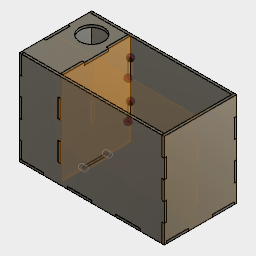
plant (Autodesk Fusion 360 design; units mm, degrees)
Autodesk Fusion 360 part; units mm, degrees
(part 1 of 2)
sketch "Sketch1" plane through (300, 0, 0) normal (1, 0, 0) x (0, 0, -1) in component "Right"
  line L0 (-145, 0) -> (-100, 0)
  line L1 (-100, 0) -> (-100, 5)
  line L2 (-100, 5) -> (-145, 5)
  line L3 (-145, 5) -> (-145, 0)
  line L4 (-50, 0) -> (-5, 0)
  line L5 (-5, 0) -> (-5, 5)
  line L6 (-5, 5) -> (-50, 5)
  line L7 (-50, 5) -> (-50, 0)
  line L8 (0, 0) -> (-150, 0)
  line L9 (-150, 0) -> (-150, 195)
  line L10 (-150, 195) -> (0, 195)
  line L11 (0, 195) -> (0, 0)
  dimension "d26" = 195
  measures "d26" distance of L8.end L9.end
extrude "Extrude1" add sketch "Sketch1" against normal blind 5 contours L1 L2 L3 L5 L6 L7 L8 L9 L10 L11 makes body 1 in component "Right"
sketch "Sketch2" plane through (300, 0, 0) normal (1, 0, 0) x (0, 0, -1) in component "Right"
  line L0 (0, 195) -> (-150, 195)
  line L1 (-150, 195) -> (-150, 0)
  line L2 (-150, 0) -> (-145, 0)
  line L3 (-145, 0) -> (-145, 5)
  line L4 (-145, 5) -> (-100, 5)
  line L5 (-100, 5) -> (-100, 0)
  line L6 (-100, 0) -> (-50, 0)
  line L7 (-50, 0) -> (-50, 5)
  line L8 (-50, 5) -> (-5, 5)
  line L9 (-5, 5) -> (-5, 0)
  line L10 (-5, 0) -> (0, 0)
  line L11 (0, 0) -> (0, 195)
  line L12 (-100, 195) -> (-100, 190)
  line L13 (-100, 190) -> (-145, 190)
  line L14 (-145, 190) -> (-145, 195)
  dimension "d29" = 5
  dimension "d30" = 45
  measures "d29" distance of L12.start L12.end
  measures "d30" distance of L12.end L13.end
extrude "Extrude2" cut sketch "Sketch2" against normal blind 5 contours L0 L12 L13 L14 bodies 1 in component "Right"
sketch "Sketch3" plane through (300, 0, 0) normal (1, 0, 0) x (0, 0, -1) in component "Right"
  line L0 (-145, 190) -> (-145, 195)
  line L1 (-145, 195) -> (-150, 195)
  line L2 (-150, 195) -> (-150, 0)
  line L3 (-150, 0) -> (-145, 0)
  line L4 (-145, 0) -> (-145, 5)
  line L5 (-145, 5) -> (-100, 5)
  line L6 (-100, 5) -> (-100, 0)
  line L7 (-100, 0) -> (-50, 0)
  line L8 (-50, 0) -> (-50, 5)
  line L9 (-50, 5) -> (-5, 5)
  line L10 (-5, 5) -> (-5, 0)
  line L11 (-5, 0) -> (0, 0)
  line L12 (0, 0) -> (0, 195)
  line L13 (0, 195) -> (-100, 195)
  line L14 (-100, 195) -> (-100, 190)
  line L15 (-100, 190) -> (-145, 190)
  line L16 (-50, 195) -> (-50, 190)
  line L17 (-50, 190) -> (-5, 190)
  line L18 (-5, 190) -> (-5, 195)
  line L19 (-50, 195) -> (-5, 195)
  dimension "d33" = 5
  dimension "d34" = 45
  measures "d33" distance of L16.start L16.end
  measures "d34" distance of L16.end L17.end
extrude "Extrude3" cut sketch "Sketch3" against normal blind 5 contours L13 L16 L17 L18 L19 bodies 1 in component "Right"
sketch "Sketch4" plane through (300, 0, 0) normal (1, 0, 0) x (0, 0, -1) in component "Right"
  line L0 (-50, 190) -> (-50, 195)
  line L1 (-50, 195) -> (-100, 195)
  line L2 (-100, 195) -> (-100, 190)
  line L3 (-100, 190) -> (-145, 190)
  line L4 (-145, 190) -> (-145, 195)
  line L5 (-145, 195) -> (-150, 195)
  line L6 (-150, 195) -> (-150, 0)
  line L7 (-150, 0) -> (-145, 0)
  line L8 (-145, 0) -> (-145, 5)
  line L9 (-145, 5) -> (-100, 5)
  line L10 (-100, 5) -> (-100, 0)
  line L11 (-100, 0) -> (-50, 0)
  line L12 (-50, 0) -> (-50, 5)
  line L13 (-50, 5) -> (-5, 5)
  line L14 (-5, 5) -> (-5, 0)
  line L15 (-5, 0) -> (0, 0)
  line L16 (0, 0) -> (0, 195)
  line L17 (0, 195) -> (-5, 195)
  line L18 (-5, 195) -> (-5, 190)
  line L19 (-5, 190) -> (-50, 190)
  line L20 (0, 0) -> (0, 39)
  line L21 (0, 39) -> (-5, 39)
  line L22 (-5, 39) -> (-5, 78)
  line L23 (-5, 78) -> (0, 78)
  dimension "d37" = 39
  dimension "d38" = 5
  dimension "d39" = 90
  dimension "d40" = 39
  dimension "d41" = 90
  dimension "d42" = 5
  measures "d37" distance of L15.end L20.end
  measures "d38" distance of L20.end L21.end
  measures "d39" angle of L21 L22
  measures "d40" distance of L21.end L22.end
  measures "d41" angle of L22 L23
  measures "d42" distance of L22.end L23.end
extrude "Extrude4" cut sketch "Sketch4" against normal blind 5 contours L16 L21 L22 L23 bodies 1 in component "Right"
sketch "Sketch5" plane through (300, 0, 0) normal (1, 0, 0) x (0, 0, -1) in component "Right"
  line L0 (0, 39) -> (-5, 39)
  line L1 (-5, 39) -> (-5, 78)
  line L2 (-5, 78) -> (0, 78)
  line L3 (0, 78) -> (0, 195)
  line L4 (0, 195) -> (-5, 195)
  line L5 (-5, 195) -> (-5, 190)
  line L6 (-5, 190) -> (-50, 190)
  line L7 (-50, 190) -> (-50, 195)
  line L8 (-50, 195) -> (-100, 195)
  line L9 (-100, 195) -> (-100, 190)
  line L10 (-100, 190) -> (-145, 190)
  line L11 (-145, 190) -> (-145, 195)
  line L12 (-145, 195) -> (-150, 195)
  line L13 (-150, 195) -> (-150, 0)
  line L14 (-150, 0) -> (-145, 0)
  line L15 (-145, 0) -> (-145, 5)
  line L16 (-145, 5) -> (-100, 5)
  line L17 (-100, 5) -> (-100, 0)
  line L18 (-100, 0) -> (-50, 0)
  line L19 (-50, 0) -> (-50, 5)
  line L20 (-50, 5) -> (-5, 5)
  line L21 (-5, 5) -> (-5, 0)
  line L22 (-5, 0) -> (0, 0)
  line L23 (0, 0) -> (0, 39)
  line L24 (0, 78) -> (0, 117)
  line L25 (0, 117) -> (-5, 117)
  line L26 (-5, 117) -> (-5, 156)
  line L27 (-5, 156) -> (0, 156)
  dimension "d45" = 39
  dimension "d46" = 5
  dimension "d47" = 90
  dimension "d48" = 39
  dimension "d49" = 90
  dimension "d50" = 5
  measures "d45" distance of L2.end L24.end
  measures "d46" distance of L24.end L25.end
  measures "d47" angle of L25 L26
  measures "d48" distance of L25.end L26.end
  measures "d49" angle of L26 L27
  measures "d50" distance of L26.end L27.end
extrude "Extrude5" cut sketch "Sketch5" against normal blind 5 contours L3 L25 L26 L27 bodies 1 in component "Right"
sketch "Sketch6" plane through (300, 0, 0) normal (1, 0, 0) x (0, 0, -1) in component "Right"
  line L0 (0, 117) -> (-5, 117)
  line L1 (-5, 117) -> (-5, 156)
  line L2 (-5, 156) -> (0, 156)
  line L3 (0, 156) -> (0, 195)
  line L4 (0, 195) -> (-5, 195)
  line L5 (-5, 195) -> (-5, 190)
  line L6 (-5, 190) -> (-50, 190)
  line L7 (-50, 190) -> (-50, 195)
  line L8 (-50, 195) -> (-100, 195)
  line L9 (-100, 195) -> (-100, 190)
  line L10 (-100, 190) -> (-145, 190)
  line L11 (-145, 190) -> (-145, 195)
  line L12 (-145, 195) -> (-150, 195)
  line L13 (-150, 195) -> (-150, 0)
  line L14 (-150, 0) -> (-145, 0)
  line L15 (-145, 0) -> (-145, 5)
  line L16 (-145, 5) -> (-100, 5)
  line L17 (-100, 5) -> (-100, 0)
  line L18 (-100, 0) -> (-50, 0)
  line L19 (-50, 0) -> (-50, 5)
  line L20 (-50, 5) -> (-5, 5)
  line L21 (-5, 5) -> (-5, 0)
  line L22 (-5, 0) -> (0, 0)
  line L23 (0, 0) -> (0, 39)
  line L24 (0, 39) -> (-5, 39)
  line L25 (-5, 39) -> (-5, 78)
  line L26 (-5, 78) -> (0, 78)
  line L27 (0, 78) -> (0, 117)
  line L28 (-150, 0) -> (-150, 39)
  line L29 (-150, 39) -> (-145, 39)
  line L30 (-145, 39) -> (-145, 78)
  line L31 (-145, 78) -> (-150, 78)
  line L32 (-150, 78) -> (-150, 117)
  line L33 (-150, 117) -> (-145, 117)
  line L34 (-145, 117) -> (-145, 156)
  line L35 (-145, 156) -> (-150, 156)
  dimension "d53" = 39
  dimension "d54" = 5
  dimension "d55" = 90
  dimension "d56" = 39
  dimension "d57" = 90
  dimension "d58" = 5
  dimension "d59" = 39
  dimension "d60" = 5
  dimension "d61" = 90
  dimension "d62" = 39
  measures "d53" distance of L13.end L28.end
  measures "d54" distance of L28.end L29.end
  measures "d55" angle of L29 L30
  measures "d56" distance of L29.end L30.end
  measures "d57" angle of L30 L31
  measures "d58" distance of L30.end L31.end
  measures "d59" distance of L31.end L32.end
  measures "d60" distance of L32.end L33.end
  measures "d61" angle of L33 L34
  measures "d62" distance of L33.end L34.end
extrude "Extrude6" cut sketch "Sketch6" against normal blind 5 contours L13 L33 L34 L35 | L13 L29 L30 L31 bodies 1 in component "Right"
sketch "Sketch7" plane through (295, 0, 0) normal (-1, 0, 0) x (0, 0, 1) in component "Right"
  line L0 (150, 117) -> (145, 117)
  line L1 (145, 117) -> (145, 156)
  line L2 (145, 156) -> (150, 156)
  line L3 (150, 156) -> (150, 195)
  line L4 (150, 195) -> (145, 195)
  line L5 (145, 195) -> (145, 190)
  line L6 (145, 190) -> (100, 190)
  line L7 (100, 190) -> (100, 195)
  line L8 (100, 195) -> (50, 195)
  line L9 (50, 195) -> (50, 190)
  line L10 (50, 190) -> (5, 190)
  line L11 (5, 190) -> (5, 195)
  line L12 (5, 195) -> (0, 195)
  line L13 (0, 195) -> (0, 156)
  line L14 (0, 156) -> (5, 156)
  line L15 (5, 156) -> (5, 117)
  line L16 (5, 117) -> (0, 117)
  line L17 (0, 117) -> (0, 78)
  line L18 (0, 78) -> (5, 78)
  line L19 (5, 78) -> (5, 39)
  line L20 (5, 39) -> (0, 39)
  line L21 (0, 39) -> (0, 0)
  line L22 (0, 0) -> (5, 0)
  line L23 (5, 0) -> (5, 5)
  line L24 (5, 5) -> (50, 5)
  line L25 (50, 5) -> (50, 0)
  line L26 (50, 0) -> (100, 0)
  line L27 (100, 0) -> (100, 5)
  line L28 (100, 5) -> (145, 5)
  line L29 (145, 5) -> (145, 0)
  line L30 (145, 0) -> (150, 0)
  line L31 (150, 0) -> (150, 39)
  line L32 (150, 39) -> (145, 39)
  line L33 (145, 39) -> (145, 78)
  line L34 (145, 78) -> (150, 78)
  line L35 (150, 78) -> (150, 117)
sketch "Sketch1 (2)" plane through (0, 0, 0) normal (-1, 0, 0) x (0, 0, 1) in component "Left"
  line L0 (100, 0) -> (150, 0)
  line L1 (150, 0) -> (150, 5)
  line L2 (150, 5) -> (100, 5)
  line L3 (100, 5) -> (100, 0)
  line L4 (0, 0) -> (50, 0)
  line L5 (50, 0) -> (50, 5)
  line L6 (50, 5) -> (0, 5)
  line L7 (0, 5) -> (0, 0)
  line L8 (150, 0) -> (0, 0)
  line L9 (0, 0) -> (0, 195)
  line L10 (0, 195) -> (150, 195)
  line L11 (150, 195) -> (150, 0)
  line L12 (100, 0) -> (100, 5)
  line L13 (100, 5) -> (145, 5)
  line L14 (145, 5) -> (145, 0)
  line L15 (5, 5) -> (5, 0)
  line L16 (150, 78) -> (145, 78)
  line L17 (145, 78) -> (145, 39)
  line L18 (145, 39) -> (150, 39)
  line L19 (150, 156) -> (145, 156)
  line L20 (145, 156) -> (145, 117)
  line L21 (145, 117) -> (150, 117)
  line L22 (100, 195) -> (100, 190)
  line L23 (100, 190) -> (145, 190)
  line L24 (145, 190) -> (145, 195)
  line L25 (50, 195) -> (50, 190)
  line L26 (50, 190) -> (5, 190)
  line L27 (5, 190) -> (5, 195)
  line L28 (0, 156) -> (5, 156)
  line L29 (5, 117) -> (0, 117)
  line L30 (5, 156) -> (5, 117)
  line L31 (0, 78) -> (5, 78)
  line L32 (5, 39) -> (0, 39)
  line L33 (5, 78) -> (5, 39)
  point P0 (0, 195)
  point P1 (145, 5)
  point P2 (145, 0)
  point P3 (5, 5)
  point P4 (5, 0)
  point P5 (150, 78)
  point P6 (145, 78)
  point P7 (145, 39)
  point P8 (150, 39)
  point P9 (150, 156)
  point P10 (145, 156)
  point P11 (145, 117)
  point P12 (150, 117)
  point P13 (100, 195)
  point P14 (100, 190)
  point P15 (145, 190)
  point P16 (145, 195)
  point P17 (50, 195)
  point P18 (50, 190)
  point P19 (5, 190)
  point P20 (5, 195)
  point P21 (0, 156)
  point P22 (5, 156)
  point P23 (5, 117)
  point P24 (0, 78)
  point P25 (5, 78)
  point P26 (5, 39)
extrude "Extrude1'" add sketch "Sketch1 (2)" against normal blind 5 separate body contours L2 L3 L5 L6 L8 L9 L10 L11 L12 L13 L16 L17 L18 L19 L20 L21 L22 L23 L24 L25 L26 L27 L28 L29 L30 L31 L32 L33 makes body 2 in component "Left"
sketch "Sketch1 (3)" plane through (0, 0, 0) normal (0, 0, -1) x (-1, 0, 0) in component "Back"
  line L0 (-250, 0) -> (-200, 0)
  line L1 (-200, 0) -> (-200, 5)
  line L2 (-200, 5) -> (-250, 5)
  line L3 (-250, 5) -> (-250, 0)
  line L4 (-150, 0) -> (-100, 0)
  line L5 (-100, 0) -> (-100, 5)
  line L6 (-100, 5) -> (-150, 5)
  line L7 (-150, 5) -> (-150, 0)
  line L8 (-50, 0) -> (0, 0)
  line L9 (0, 0) -> (0, 5)
  line L10 (0, 5) -> (-50, 5)
  line L11 (-50, 5) -> (-50, 0)
  line L12 (0, 5) -> (0, 39)
  line L13 (0, 39) -> (-5, 39)
  line L14 (-5, 39) -> (-5, 5)
  line L15 (-5, 5) -> (0, 5)
  line L16 (0, 78) -> (0, 117)
  line L17 (0, 117) -> (-5, 117)
  line L18 (-5, 117) -> (-5, 78)
  line L19 (-5, 78) -> (0, 78)
  line L20 (0, 156) -> (0, 195)
  line L21 (0, 195) -> (-5, 195)
  line L22 (-5, 195) -> (-5, 156)
  line L23 (-5, 156) -> (0, 156)
  line L24 (-300, 156) -> (-295, 156)
  line L25 (-295, 156) -> (-295, 195)
  line L26 (-295, 195) -> (-300, 195)
  line L27 (-300, 195) -> (-300, 156)
  line L28 (-295, 117) -> (-300, 117)
  line L29 (-300, 117) -> (-300, 78)
  line L30 (-300, 78) -> (-295, 78)
  line L31 (-295, 78) -> (-295, 117)
  line L32 (-295, 39) -> (-300, 39)
  line L33 (-300, 39) -> (-300, 0)
  line L34 (-300, 0) -> (-295, 0)
  line L35 (-295, 0) -> (-295, 39)
  line L36 (-300, 195) -> (0, 195)
  line L37 (0, 195) -> (0, 0)
  line L38 (0, 0) -> (-300, 0)
  line L39 (-300, 0) -> (-300, 195)
extrude "Extrude1''" add sketch "Sketch1 (3)" against normal blind 5 separate body contours L1 L2 L3 L5 L6 L7 L10 L11 L13 L14 L17 L18 L19 L22 L23 L24 L25 L28 L30 L31 L32 L35 L36 L37 L38 L39 makes body 3 in component "Back"
sketch "Sketch1 (4)" plane through (0, 0, 150) normal (0, 0, 1) x (1, 0, 0) in component "Front"
  line L0 (0, 0) -> (50, 0)
  line L1 (50, 0) -> (50, 5)
  line L2 (50, 5) -> (0, 5)
  line L3 (0, 5) -> (0, 0)
  line L4 (100, 0) -> (150, 0)
  line L5 (150, 0) -> (150, 5)
  line L6 (150, 5) -> (100, 5)
  line L7 (100, 5) -> (100, 0)
  line L8 (200, 0) -> (250, 0)
  line L9 (250, 0) -> (250, 5)
  line L10 (250, 5) -> (200, 5)
  line L11 (200, 5) -> (200, 0)
  line L12 (295, 156) -> (300, 156)
  line L13 (300, 156) -> (300, 195)
  line L14 (300, 195) -> (295, 195)
  line L15 (295, 195) -> (295, 156)
  line L16 (300, 117) -> (295, 117)
  line L17 (295, 117) -> (295, 78)
  line L18 (295, 78) -> (300, 78)
  line L19 (300, 78) -> (300, 117)
  line L20 (300, 39) -> (295, 39)
  line L21 (295, 39) -> (295, 0)
  line L22 (295, 0) -> (300, 0)
  line L23 (300, 0) -> (300, 39)
  line L24 (0, 39) -> (0, 5)
  line L25 (0, 5) -> (5, 5)
  line L26 (5, 5) -> (5, 39)
  line L27 (5, 39) -> (0, 39)
  line L28 (0, 117) -> (0, 78)
  line L29 (0, 78) -> (5, 78)
  line L30 (5, 78) -> (5, 117)
  line L31 (5, 117) -> (0, 117)
  line L32 (0, 195) -> (0, 156)
  line L33 (0, 156) -> (5, 156)
  line L34 (5, 156) -> (5, 195)
  line L35 (5, 195) -> (0, 195)
  line L36 (0, 195) -> (300, 195)
  line L37 (300, 195) -> (300, 0)
  line L38 (300, 0) -> (0, 0)
  line L39 (0, 0) -> (0, 195)
extrude "Extrude1'''" add sketch "Sketch1 (4)" against normal blind 5 separate body contours L1 L2 L5 L6 L7 L9 L10 L11 L12 L15 L16 L17 L18 L20 L21 L26 L27 L29 L30 L31 L33 L34 L36 L37 L38 L39 makes body 4 in component "Front"
sketch "Sketch2 (2)" plane through (300, 0, 0) normal (1, 0, 0) x (0, 0, -1) in component "Back"
  line L0 (-150, 156) -> (-145, 156)
  line L1 (-145, 156) -> (-145, 117)
  line L2 (-145, 117) -> (-150, 117)
  line L3 (-150, 117) -> (-150, 78)
  line L4 (-150, 78) -> (-145, 78)
  line L5 (-145, 78) -> (-145, 39)
  line L6 (-145, 39) -> (-150, 39)
  line L7 (-150, 39) -> (-150, 0)
  line L8 (-150, 0) -> (-145, 0)
  line L9 (-145, 0) -> (-145, 5)
  line L10 (-145, 5) -> (-100, 5)
  line L11 (-100, 5) -> (-100, 0)
  line L12 (-100, 0) -> (-50, 0)
  line L13 (-50, 0) -> (-50, 5)
  line L14 (-50, 5) -> (-5, 5)
  line L15 (-5, 5) -> (-5, 0)
  line L16 (-5, 0) -> (0, 0)
  line L17 (0, 0) -> (0, 39)
  line L18 (0, 39) -> (-5, 39)
  line L19 (-5, 39) -> (-5, 78)
  line L20 (-5, 78) -> (0, 78)
  line L21 (0, 78) -> (0, 117)
  line L22 (0, 117) -> (-5, 117)
  line L23 (-5, 117) -> (-5, 156)
  line L24 (-5, 156) -> (0, 156)
  line L25 (0, 156) -> (0, 195)
  line L26 (0, 195) -> (-5, 195)
  line L27 (-5, 195) -> (-5, 190)
  line L28 (-5, 190) -> (-50, 190)
  line L29 (-50, 190) -> (-50, 195)
  line L30 (-50, 195) -> (-100, 195)
  line L31 (-100, 195) -> (-100, 190)
  line L32 (-100, 190) -> (-145, 190)
  line L33 (-145, 190) -> (-145, 195)
  line L34 (-145, 195) -> (-150, 195)
  line L35 (-150, 195) -> (-150, 156)
sketch "Sketch3 (2)" plane through (0, 0, 5) normal (0, 0, 1) x (1, 0, 0) in component "Back"
  line L0 (295, 0) -> (295, 39)
  line L1 (295, 39) -> (300, 39)
  line L2 (300, 39) -> (300, 78)
  line L3 (300, 78) -> (295, 78)
  line L4 (295, 78) -> (295, 117)
  line L5 (295, 117) -> (300, 117)
  line L6 (300, 117) -> (300, 156)
  line L7 (300, 156) -> (295, 156)
  line L8 (295, 156) -> (295, 195)
  line L9 (295, 195) -> (5, 195)
  line L10 (5, 195) -> (5, 156)
  line L11 (5, 156) -> (0, 156)
  line L12 (0, 156) -> (0, 117)
  line L13 (0, 117) -> (5, 117)
  line L14 (5, 117) -> (5, 78)
  line L15 (5, 78) -> (0, 78)
  line L16 (0, 78) -> (0, 39)
  line L17 (0, 39) -> (5, 39)
  line L18 (5, 39) -> (5, 5)
  line L19 (5, 5) -> (50, 5)
  line L20 (50, 5) -> (50, 0)
  line L21 (50, 0) -> (100, 0)
  line L22 (100, 0) -> (100, 5)
  line L23 (100, 5) -> (150, 5)
  line L24 (150, 5) -> (150, 0)
  line L25 (150, 0) -> (200, 0)
  line L26 (200, 0) -> (200, 5)
  line L27 (200, 5) -> (250, 5)
  line L28 (250, 5) -> (250, 0)
  line L29 (250, 0) -> (295, 0)
  line L30 (80, 39) -> (85, 39)
  line L31 (85, 39) -> (85, 78)
  line L32 (85, 78) -> (80, 78)
  line L33 (80, 78) -> (80, 39)
  line L34 (85, 156) -> (80, 156)
  line L35 (80, 156) -> (85, 156)
  line L36 (85, 156) -> (85, 117)
  line L37 (85, 117) -> (80, 117)
  line L38 (80, 117) -> (80, 156)
  dimension "d76" = 75
  dimension "d77" = 5
  dimension "d78" = 39
  dimension "d79" = 39
  dimension "d82" = 5
  dimension "d83" = 39
  measures "d76" distance of L18 L33
  measures "d77" distance of L31.end L32.end
  measures "d78" distance of L20.end L30.start
  measures "d79" distance of L30.start L32.end
  measures "d82" distance of L34.end L34.start
  measures "d83" distance of L34.end L37.end
extrude "Extrude2'" cut sketch "Sketch3 (2)" against normal blind 5 contours L30 L31 L32 L33 | L34 L35 L36 L37 L38 bodies 3 in component "Back"
sketch "Sketch2 (3)" plane through (0, 0, 145) normal (0, 0, -1) x (-1, 0, 0) in component "Front"
  line L0 (-50, 0) -> (-50, 5)
  line L1 (-50, 5) -> (-5, 5)
  line L2 (-5, 5) -> (-5, 39)
  line L3 (-5, 39) -> (0, 39)
  line L4 (0, 39) -> (0, 78)
  line L5 (0, 78) -> (-5, 78)
  line L6 (-5, 78) -> (-5, 117)
  line L7 (-5, 117) -> (0, 117)
  line L8 (0, 117) -> (0, 156)
  line L9 (0, 156) -> (-5, 156)
  line L10 (-5, 156) -> (-5, 195)
  line L11 (-5, 195) -> (-295, 195)
  line L12 (-295, 195) -> (-295, 156)
  line L13 (-295, 156) -> (-300, 156)
  line L14 (-300, 156) -> (-300, 117)
  line L15 (-300, 117) -> (-295, 117)
  line L16 (-295, 117) -> (-295, 78)
  line L17 (-295, 78) -> (-300, 78)
  line L18 (-300, 78) -> (-300, 39)
  line L19 (-300, 39) -> (-295, 39)
  line L20 (-295, 39) -> (-295, 0)
  line L21 (-295, 0) -> (-250, 0)
  line L22 (-250, 0) -> (-250, 5)
  line L23 (-250, 5) -> (-200, 5)
  line L24 (-200, 5) -> (-200, 0)
  line L25 (-200, 0) -> (-150, 0)
  line L26 (-150, 0) -> (-150, 5)
  line L27 (-150, 5) -> (-100, 5)
  line L28 (-100, 5) -> (-100, 0)
  line L29 (-100, 0) -> (-50, 0)
  line L30 (-80, 39) -> (-85, 39)
  line L31 (-85, 39) -> (-85, 78)
  line L32 (-85, 78) -> (-80, 78)
  line L33 (-80, 78) -> (-80, 39)
  line L34 (-85, 117) -> (-80, 117)
  line L35 (-80, 117) -> (-80, 156)
  line L36 (-80, 156) -> (-85, 156)
  line L37 (-85, 156) -> (-85, 117)
  dimension "d86" = 39
  dimension "d87" = 39
  dimension "d88" = 5
  dimension "d89" = 75
  dimension "d90" = 39
  dimension "d91" = 39
  dimension "d92" = 39
  measures "d86" distance of L29 L30
  measures "d87" distance of L30.start L32
  measures "d88" distance of L31.end L32.end
  measures "d89" distance of L2.end L30.start
  measures "d90" distance of L32 L34
  measures "d91" distance of L34 L36
  measures "d92" distance of L11 L36
extrude "Extrude2''" cut sketch "Sketch2 (3)" against normal blind 5 contours L30 L31 L32 L33 | L34 L35 L36 L37 bodies 4 in component "Front"
sketch "Sketch1 (5)" plane through (0, 5, 0) normal (0, 1, 0) x (-1, 0, 0) in component "Divider2"
  line L0 (-85, 50) -> (-85, 100)
  line L1 (-85, 100) -> (-80, 100)
  line L2 (-80, 100) -> (-80, 50)
  line L3 (-80, 50) -> (-85, 50)
  line L4 (-100, 0) -> (-100, 5)
  line L5 (-100, 5) -> (-50, 5)
  line L6 (-50, 5) -> (-50, 0)
  line L7 (-50, 0) -> (0, 0)
  line L8 (0, 0) -> (0, 50)
  line L9 (0, 50) -> (-5, 50)
  line L10 (-5, 50) -> (-5, 100)
  line L11 (-5, 100) -> (0, 100)
  line L12 (0, 100) -> (0, 150)
  line L13 (0, 150) -> (-50, 150)
  line L14 (-50, 150) -> (-50, 145)
  line L15 (-50, 145) -> (-100, 145)
  line L16 (-100, 145) -> (-100, 150)
  line L17 (-100, 150) -> (-150, 150)
  line L18 (-150, 150) -> (-150, 145)
  line L19 (-150, 145) -> (-200, 145)
  line L20 (-200, 145) -> (-200, 150)
  line L21 (-200, 150) -> (-250, 150)
  line L22 (-250, 150) -> (-250, 145)
  line L23 (-250, 145) -> (-300, 145)
  line L24 (-300, 145) -> (-300, 100)
  line L25 (-300, 100) -> (-295, 100)
  line L26 (-295, 100) -> (-295, 50)
  line L27 (-295, 50) -> (-300, 50)
  line L28 (-300, 50) -> (-300, 5)
  line L29 (-300, 5) -> (-250, 5)
  line L30 (-250, 5) -> (-250, 0)
  line L31 (-250, 0) -> (-200, 0)
  line L32 (-200, 0) -> (-200, 5)
  line L33 (-200, 5) -> (-150, 5)
  line L34 (-150, 5) -> (-150, 0)
  line L35 (-150, 0) -> (-100, 0)
  line L36 (-80, 5) -> (-85, 5)
  line L37 (-85, 5) -> (-85, 145)
  line L38 (-85, 145) -> (-80, 145)
  line L39 (-80, 145) -> (-80, 5)
  point P0 (-80, 5)
  point P1 (-85, 145)
extrude "Extrude1''''" add sketch "Sketch1 (5)" along normal blind 190 separate body contours L0 L1 L2 L3 L37 L39 | L3 L5 L36 L37 L39 | L1 L15 L37 L38 L39 makes body 5 in component "Divider2"
sketch "Sketch3 (3)" plane through (0, 0, 5) normal (0, 0, -1) x (-1, 0, 0) in component "Front"
  line L0 (-85, 5) -> (-80, 5)
  line L1 (-80, 5) -> (-80, 195)
  line L2 (-80, 195) -> (-85, 195)
  line L3 (-85, 195) -> (-85, 5)
  line L4 (-85, 156) -> (-80, 156)
  line L5 (-80, 156) -> (-80, 117)
  line L6 (-80, 117) -> (-85, 117)
  line L7 (-85, 117) -> (-85, 156)
  line L8 (-85, 78) -> (-80, 78)
  line L9 (-80, 78) -> (-80, 39)
  line L10 (-80, 39) -> (-85, 39)
  line L11 (-85, 39) -> (-85, 78)
  point P0 (-85, 156)
  point P1 (-80, 117)
  point P2 (-85, 78)
  point P3 (-80, 39)
sketch "Sketch2 (4)" plane through (0, 0, 5) normal (0, 0, -1) x (-1, 0, 0) in component "Divider2"
  line L0 (-85, 5) -> (-80, 5)
  line L1 (-80, 5) -> (-80, 195)
  line L2 (-80, 195) -> (-85, 195)
  line L3 (-85, 195) -> (-85, 5)
  line L4 (-85, 156) -> (-80, 156)
  line L5 (-80, 156) -> (-80, 117)
  line L6 (-80, 117) -> (-85, 117)
  line L7 (-85, 117) -> (-85, 156)
  line L8 (-85, 78) -> (-80, 78)
  line L9 (-80, 78) -> (-80, 39)
  line L10 (-80, 39) -> (-85, 39)
  line L11 (-85, 39) -> (-85, 78)
  point P0 (-85, 156)
  point P1 (-80, 117)
  point P2 (-85, 78)
  point P3 (-80, 39)
extrude "Extrude2'''" add sketch "Sketch2 (4)" along normal blind 5 contours L1 L3 L8 L9 L10 L11 | L1 L3 L4 L5 L6 L7 bodies 5 in component "Divider2"
sketch "Sketch3 (4)" plane through (0, 0, 145) normal (0, 0, 1) x (1, 0, 0) in component "Divider2"
  line L0 (80, 5) -> (85, 5)
  line L1 (85, 5) -> (85, 195)
  line L2 (85, 195) -> (80, 195)
  line L3 (80, 195) -> (80, 5)
  line L4 (80, 156) -> (85, 156)
  line L5 (85, 156) -> (85, 117)
  line L6 (85, 117) -> (80, 117)
  line L7 (80, 117) -> (80, 156)
  line L8 (80, 78) -> (85, 78)
  line L9 (85, 78) -> (85, 39)
  line L10 (85, 39) -> (80, 39)
  line L11 (80, 39) -> (80, 78)
  point P0 (80, 156)
  point P1 (85, 117)
  point P2 (80, 78)
  point P3 (85, 39)
extrude "Extrude3'" add sketch "Sketch3 (4)" along normal blind 5 contours L1 L3 L8 L9 L10 L11 | L1 L3 L4 L5 L6 L7 bodies 5 in component "Divider2"
sketch "Sketch2 (5)" plane through (0, 5, 0) normal (0, -1, 0) x (1, 0, 0) in component "Left"
  line L0 (85, 145) -> (80, 145)
  line L1 (80, 145) -> (80, 5)
  line L2 (80, 5) -> (85, 5)
  line L3 (85, 5) -> (85, 145)
  line L4 (80, 100) -> (85, 100)
  line L5 (85, 100) -> (85, 50)
  line L6 (85, 50) -> (80, 50)
  line L7 (80, 50) -> (80, 100)
  line L8 (80, 50) -> (85, 50)
  line L9 (85, 50) -> (85, 100)
  line L10 (85, 100) -> (80, 100)
  line L11 (80, 100) -> (80, 50)
sketch "Sketch4 (2)" plane through (0, 5, 0) normal (0, -1, 0) x (1, 0, 0) in component "Divider2"
  line L0 (85, 145) -> (80, 145)
  line L1 (80, 145) -> (80, 5)
  line L2 (80, 5) -> (85, 5)
  line L3 (85, 5) -> (85, 145)
  line L4 (80, 100) -> (85, 100)
  line L5 (85, 100) -> (85, 50)
  line L6 (85, 50) -> (80, 50)
  line L7 (80, 50) -> (80, 100)
extrude "Extrude4'" add sketch "Sketch4 (2)" along normal blind 5 contours L1 L3 L4 L5 L6 L7 bodies 5 in component "Divider2"
sketch "Sketch3 (5)" plane through (0, 0, 0) normal (-1, 0, 0) x (0, 0, 1) in component "Left"
  line L0 (0, 78) -> (5, 78)
  line L1 (5, 78) -> (5, 39)
  line L2 (5, 39) -> (0, 39)
  line L3 (0, 39) -> (0, 5)
  line L4 (0, 5) -> (50, 5)
  line L5 (50, 5) -> (50, 0)
  line L6 (50, 0) -> (100, 0)
  line L7 (100, 0) -> (100, 5)
  line L8 (100, 5) -> (150, 5)
  line L9 (150, 5) -> (150, 39)
  line L10 (150, 39) -> (145, 39)
  line L11 (145, 39) -> (145, 78)
  line L12 (145, 78) -> (150, 78)
  line L13 (150, 78) -> (150, 117)
  line L14 (150, 117) -> (145, 117)
  line L15 (145, 117) -> (145, 156)
  line L16 (145, 156) -> (150, 156)
  line L17 (150, 156) -> (150, 195)
  line L18 (150, 195) -> (145, 195)
  line L19 (145, 195) -> (145, 190)
  line L20 (145, 190) -> (100, 190)
  line L21 (100, 190) -> (100, 195)
  line L22 (100, 195) -> (50, 195)
  line L23 (50, 195) -> (50, 190)
  line L24 (50, 190) -> (5, 190)
  line L25 (5, 190) -> (5, 195)
  line L26 (5, 195) -> (0, 195)
  line L27 (0, 195) -> (0, 156)
  line L28 (0, 156) -> (5, 156)
  line L29 (5, 156) -> (5, 117)
  line L30 (5, 117) -> (0, 117)
  line L31 (0, 117) -> (0, 78)
  line L32 (80, 117) -> (85, 117)
  line L33 (85, 117) -> (85, 78)
  line L34 (85, 78) -> (80, 78)
  line L35 (80, 78) -> (80, 117)
  line L36 (5, 156) -> (5, 117)
  dimension "d103" = 5
  dimension "d104" = 39
  dimension "d105" = 75
  dimension "d106" = 78
  measures "d103" distance of L32.start L32.end
  measures "d104" distance of L32.start L34.end
  measures "d105" distance of L35 L36
  measures "d106" distance of L6 L34
extrude "Extrude2''''" cut sketch "Sketch3 (5)" against normal blind 5 contours L32 L33 L34 L35 bodies 2 in component "Left"
sketch "Sketch5 (2)" plane through (80, 0, 0) normal (-1, 0, 0) x (0, 0, 1) in component "Divider2"
  line L0 (100, 5) -> (145, 5)
  line L1 (145, 5) -> (145, 39)
  line L2 (145, 39) -> (150, 39)
  line L3 (150, 39) -> (150, 78)
  line L4 (150, 78) -> (145, 78)
  line L5 (145, 78) -> (145, 117)
  line L6 (145, 117) -> (150, 117)
  line L7 (150, 117) -> (150, 156)
  line L8 (150, 156) -> (145, 156)
  line L9 (145, 156) -> (145, 195)
  line L10 (145, 195) -> (5, 195)
  line L11 (5, 195) -> (5, 156)
  line L12 (5, 156) -> (0, 156)
  line L13 (0, 156) -> (0, 117)
  line L14 (0, 117) -> (5, 117)
  line L15 (5, 117) -> (5, 78)
  line L16 (5, 78) -> (0, 78)
  line L17 (0, 78) -> (0, 39)
  line L18 (0, 39) -> (5, 39)
  line L19 (5, 39) -> (5, 5)
  line L20 (5, 5) -> (50, 5)
  line L21 (50, 5) -> (50, 0)
  line L22 (50, 0) -> (100, 0)
  line L23 (100, 0) -> (100, 5)
  line L24 (85, 117) -> (80, 117)
  line L25 (80, 117) -> (80, 78)
  line L26 (80, 78) -> (85, 78)
  line L27 (85, 78) -> (85, 117)
  dimension "d109" = 39
  dimension "d110" = 5
  dimension "d111" = 75
  dimension "d113" = 78
  measures "d109" distance of L24.start L26.end
  measures "d110" distance of L24.start L24.end
  measures "d111" distance of L15 L25
  measures "d113" distance of L10 L24
sketch "Sketch4 (3)" plane through (0, 0, 0) normal (-1, 0, 0) x (0, 0, 1) in component "Left"
  line L0 (85, 117) -> (85, 78)
  line L1 (85, 78) -> (80, 78)
  line L2 (80, 78) -> (80, 117)
  line L3 (80, 117) -> (85, 117)
  line L4 (0, 78) -> (5, 78)
  line L5 (5, 78) -> (5, 39)
  line L6 (5, 39) -> (0, 39)
  line L7 (0, 39) -> (0, 5)
  line L8 (0, 5) -> (50, 5)
  line L9 (50, 5) -> (50, 0)
  line L10 (50, 0) -> (100, 0)
  line L11 (100, 0) -> (100, 5)
  line L12 (100, 5) -> (150, 5)
  line L13 (150, 5) -> (150, 39)
  line L14 (150, 39) -> (145, 39)
  line L15 (145, 39) -> (145, 78)
  line L16 (145, 78) -> (150, 78)
  line L17 (150, 78) -> (150, 117)
  line L18 (150, 117) -> (145, 117)
  line L19 (145, 117) -> (145, 156)
  line L20 (145, 156) -> (150, 156)
  line L21 (150, 156) -> (150, 195)
  line L22 (150, 195) -> (145, 195)
  line L23 (145, 195) -> (145, 190)
  line L24 (145, 190) -> (100, 190)
  line L25 (100, 190) -> (100, 195)
  line L26 (100, 195) -> (50, 195)
  line L27 (50, 195) -> (50, 190)
  line L28 (50, 190) -> (5, 190)
  line L29 (5, 190) -> (5, 195)
  line L30 (5, 195) -> (0, 195)
  line L31 (0, 195) -> (0, 156)
  line L32 (0, 156) -> (5, 156)
  line L33 (5, 156) -> (5, 117)
  line L34 (5, 117) -> (0, 117)
  line L35 (0, 117) -> (0, 78)
  line L36 (5, 156) -> (5, 117)
  dimension "d112" = 75
  measures "d112" distance of L2 L36
extrude "Extrude5'" cut sketch "Sketch5 (2)" against normal blind 5 contours L24 L25 L26 L27 bodies 5 in component "Divider2"
extrude "Extrude3''" add sketch "Sketch4 (3)" against normal blind 5 contours L0 L1 L2 L3 bodies 2 in component "Left"
sketch "Sketch5 (3)" plane through (0, 0, 0) normal (-1, 0, 0) x (0, 0, 1) in component "Left"
  line L0 (0, 78) -> (5, 78)
  line L1 (5, 78) -> (5, 39)
  line L2 (5, 39) -> (0, 39)
  line L3 (0, 39) -> (0, 5)
  line L4 (0, 5) -> (50, 5)
  line L5 (50, 5) -> (50, 0)
  line L6 (50, 0) -> (100, 0)
  line L7 (100, 0) -> (100, 5)
  line L8 (100, 5) -> (150, 5)
  line L9 (150, 5) -> (150, 39)
  line L10 (150, 39) -> (145, 39)
  line L11 (145, 39) -> (145, 78)
  line L12 (145, 78) -> (150, 78)
  line L13 (150, 78) -> (150, 117)
  line L14 (150, 117) -> (145, 117)
  line L15 (145, 117) -> (145, 156)
  line L16 (145, 156) -> (150, 156)
  line L17 (150, 156) -> (150, 195)
  line L18 (150, 195) -> (145, 195)
  line L19 (145, 195) -> (145, 190)
  line L20 (145, 190) -> (100, 190)
  line L21 (100, 190) -> (100, 195)
  line L22 (100, 195) -> (50, 195)
  line L23 (50, 195) -> (50, 190)
  line L24 (50, 190) -> (5, 190)
  line L25 (5, 190) -> (5, 195)
  line L26 (5, 195) -> (0, 195)
  line L27 (0, 195) -> (0, 156)
  line L28 (0, 156) -> (5, 156)
  line L29 (5, 156) -> (5, 117)
  line L30 (5, 117) -> (0, 117)
  line L31 (0, 117) -> (0, 78)
  line L32 (80, 117) -> (85, 117)
  line L33 (85, 117) -> (85, 78)
  line L34 (85, 78) -> (80, 78)
  line L35 (80, 78) -> (80, 117)
  line L36 (5, 156) -> (5, 117)
  dimension "d118" = 5
  dimension "d119" = 75
  dimension "d120" = 78
  dimension "d121" = 39
  measures "d118" distance of L32.start L32.end
  measures "d119" distance of L35 L36
  measures "d120" distance of L22 L32
  measures "d121" distance of L32.end L33.end
extrude "Extrude4''" cut sketch "Sketch5 (3)" against normal blind 5 contours L32 L33 L34 L35 bodies 2 in component "Left"
sketch "Sketch1 (6)" plane through (0, 0, 0) normal (0, -1, 0) x (1, 0, 0) in component "Base"
  line L0 (300, 50) -> (300, 100)
  line L1 (300, 100) -> (295, 100)
  line L2 (295, 100) -> (295, 50)
  line L3 (295, 50) -> (300, 50)
  line L4 (300, 145) -> (300, 150)
  line L5 (300, 150) -> (295, 150)
  line L6 (295, 150) -> (295, 145)
  line L7 (295, 145) -> (300, 145)
  line L8 (300, 0) -> (300, 5)
  line L9 (300, 5) -> (295, 5)
  line L10 (295, 5) -> (295, 0)
  line L11 (295, 0) -> (300, 0)
  line L12 (295, 150) -> (250, 150)
  line L13 (250, 150) -> (250, 145)
  line L14 (250, 145) -> (295, 145)
  line L15 (295, 145) -> (295, 150)
  line L16 (200, 150) -> (150, 150)
  line L17 (150, 150) -> (150, 145)
  line L18 (150, 145) -> (200, 145)
  line L19 (200, 145) -> (200, 150)
  line L20 (100, 150) -> (50, 150)
  line L21 (50, 150) -> (50, 145)
  line L22 (50, 145) -> (100, 145)
  line L23 (100, 145) -> (100, 150)
  line L24 (50, 0) -> (100, 0)
  line L25 (100, 0) -> (100, 5)
  line L26 (100, 5) -> (50, 5)
  line L27 (50, 5) -> (50, 0)
  line L28 (150, 0) -> (200, 0)
  line L29 (200, 0) -> (200, 5)
  line L30 (200, 5) -> (150, 5)
  line L31 (150, 5) -> (150, 0)
  line L32 (250, 0) -> (295, 0)
  line L33 (295, 0) -> (295, 5)
  line L34 (295, 5) -> (250, 5)
  line L35 (250, 5) -> (250, 0)
  line L36 (295, 150) -> (295, 145)
  line L37 (295, 145) -> (295, 150)
  line L38 (295, 150) -> (295, 145)
  line L39 (295, 145) -> (295, 100)
  line L40 (295, 100) -> (295, 50)
  line L41 (295, 50) -> (295, 5)
  line L42 (295, 5) -> (295, 0)
  line L43 (295, 0) -> (295, 5)
  line L44 (295, 5) -> (295, 0)
  line L45 (295, 0) -> (295, 5)
  line L46 (295, 5) -> (295, 0)
  line L47 (295, 0) -> (295, 5)
  line L48 (295, 5) -> (295, 50)
  line L49 (295, 50) -> (295, 100)
  line L50 (295, 100) -> (295, 145)
  line L51 (295, 145) -> (295, 150)
  line L52 (295, 150) -> (295, 145)
  line L53 (295, 145) -> (295, 150)
  line L54 (300, 100) -> (300, 50)
  line L55 (80, 50) -> (85, 50)
  line L56 (85, 50) -> (85, 100)
  line L57 (85, 100) -> (80, 100)
  line L58 (80, 100) -> (80, 50)
  line L59 (0, 100) -> (0, 50)
  line L60 (0, 50) -> (5, 50)
  line L61 (5, 50) -> (5, 100)
  line L62 (5, 100) -> (0, 100)
  line L63 (0, 150) -> (300, 150)
  line L64 (300, 150) -> (300, 0)
  line L65 (300, 0) -> (0, 0)
  line L66 (0, 0) -> (0, 150)
  point P0 (0, 150)
extrude "Extrude1'''''" add sketch "Sketch1 (6)" against normal blind 5 separate body contours L3 L9 L41 L48 L64 | L1 L7 L39 L50 L64 | L2 L13 L14 L17 L18 L19 L21 L22 L23 L25 L26 L27 L29 L30 L31 L34 L35 L39 L40 L41 L48 L49 L50 L60 L61 L62 L63 L65 L66 makes body 6 in component "Base"
sketch "Sketch2 (6)" plane through (0, 5, 0) normal (0, 1, 0) x (-1, 0, 0) in component "Base"
  line L0 (-80, 100) -> (-80, 50)
  line L1 (-80, 50) -> (-85, 50)
  line L2 (-85, 50) -> (-85, 100)
  line L3 (-85, 100) -> (-80, 100)
  line L4 (-295, 100) -> (-295, 50)
  line L5 (-295, 50) -> (-300, 50)
  line L6 (-300, 50) -> (-300, 5)
  line L7 (-300, 5) -> (-250, 5)
  line L8 (-250, 5) -> (-250, 0)
  line L9 (-250, 0) -> (-200, 0)
  line L10 (-200, 0) -> (-200, 5)
  line L11 (-200, 5) -> (-150, 5)
  line L12 (-150, 5) -> (-150, 0)
  line L13 (-150, 0) -> (-100, 0)
  line L14 (-100, 0) -> (-100, 5)
  line L15 (-100, 5) -> (-50, 5)
  line L16 (-50, 5) -> (-50, 0)
  line L17 (-50, 0) -> (0, 0)
  line L18 (0, 0) -> (0, 50)
  line L19 (0, 50) -> (-5, 50)
  line L20 (-5, 50) -> (-5, 100)
  line L21 (-5, 100) -> (0, 100)
  line L22 (0, 100) -> (0, 150)
  line L23 (0, 150) -> (-50, 150)
  line L24 (-50, 150) -> (-50, 145)
  line L25 (-50, 145) -> (-100, 145)
  line L26 (-100, 145) -> (-100, 150)
  line L27 (-100, 150) -> (-150, 150)
  line L28 (-150, 150) -> (-150, 145)
  line L29 (-150, 145) -> (-200, 145)
  line L30 (-200, 145) -> (-200, 150)
  line L31 (-200, 150) -> (-250, 150)
  line L32 (-250, 150) -> (-250, 145)
  line L33 (-250, 145) -> (-300, 145)
  line L34 (-300, 145) -> (-300, 100)
  line L35 (-300, 100) -> (-295, 100)
  line L36 (-17.5, 80) -> (-67.5, 80)
  line L37 (-67.5, 80) -> (-67.5, 85)
  line L38 (-67.5, 85) -> (-17.5, 85)
  line L39 (-17.5, 85) -> (-17.5, 80)
  line L40 (-5, 5) -> (-5, 50)
  line L41 (-80, 145) -> (-80, 5)
  dimension "d126" = 50
  dimension "d127" = 75
  dimension "d128" = 12.5
  measures "d126" distance of L36.start L36.end
  measures "d127" distance of L40 L41
  measures "d128" distance of L20 L39
extrude "Extrude2'''''" cut sketch "Sketch2 (6)" against normal blind 5 contours L36 L37 L38 L39 bodies 6 in component "Base"
sketch "Sketch1 (7)" plane through (0, 0, 5) normal (0, 0, 1) x (1, 0, 0) in component "Divider4"
  line L0 (85, 156) -> (85, 117)
  line L1 (85, 117) -> (80, 117)
  line L2 (80, 117) -> (80, 156)
  line L3 (80, 156) -> (85, 156)
  line L4 (85, 39) -> (80, 39)
  line L5 (80, 39) -> (80, 78)
  line L6 (80, 78) -> (85, 78)
  line L7 (85, 78) -> (85, 39)
  line L8 (295, 0) -> (295, 39)
  line L9 (295, 39) -> (300, 39)
  line L10 (300, 39) -> (300, 78)
  line L11 (300, 78) -> (295, 78)
  line L12 (295, 78) -> (295, 117)
  line L13 (295, 117) -> (300, 117)
  line L14 (300, 117) -> (300, 156)
  line L15 (300, 156) -> (295, 156)
  line L16 (295, 156) -> (295, 195)
  line L17 (295, 195) -> (5, 195)
  line L18 (5, 195) -> (5, 156)
  line L19 (5, 156) -> (0, 156)
  line L20 (0, 156) -> (0, 117)
  line L21 (0, 117) -> (5, 117)
  line L22 (5, 117) -> (5, 78)
  line L23 (5, 78) -> (0, 78)
  line L24 (0, 78) -> (0, 39)
  line L25 (0, 39) -> (5, 39)
  line L26 (5, 39) -> (5, 5)
  line L27 (5, 5) -> (50, 5)
  line L28 (50, 5) -> (50, 0)
  line L29 (50, 0) -> (100, 0)
  line L30 (100, 0) -> (100, 5)
  line L31 (100, 5) -> (150, 5)
  line L32 (150, 5) -> (150, 0)
  line L33 (150, 0) -> (200, 0)
  line L34 (200, 0) -> (200, 5)
  line L35 (200, 5) -> (250, 5)
  line L36 (250, 5) -> (250, 0)
  line L37 (250, 0) -> (295, 0)
sketch "Sketch2 (7)" plane through (0, 0, 5) normal (0, 0, 1) x (1, 0, 0) in component "Divider4"
  line L0 (5, 195) -> (80, 195)
  line L1 (80, 195) -> (80, 5)
  line L2 (80, 5) -> (5, 5)
  line L3 (5, 5) -> (5, 195)
  point P0 (5, 195)
  point P1 (80, 5)
extrude "Extrude1''''''" add sketch "Sketch2 (7)" along normal blind 5 separate body makes body 7 in component "Divider4"
sketch "Sketch6 (2)" plane through (5, 0, -75) normal (-1, 0, 0) x (0, 0, 1) in component "Divider2"
  line L0 (80, 195) -> (80, 5)
  line L1 (80, 5) -> (85, 5)
  line L2 (85, 5) -> (85, 195)
  line L3 (85, 195) -> (80, 195)
sketch "Sketch3 (6)" plane through (80, 0, -75) normal (1, 0, 0) x (0, 0, -1) in component "Divider4"
  line L0 (-80, 5) -> (-80, 195)
  line L1 (-80, 195) -> (-85, 195)
  line L2 (-85, 195) -> (-85, 5)
  line L3 (-85, 5) -> (-80, 5)
  line L4 (-80, 117) -> (-85, 117)
  line L5 (-85, 117) -> (-85, 78)
  line L6 (-85, 78) -> (-80, 78)
  line L7 (-80, 78) -> (-80, 117)
  point P0 (-80, 117)
  dimension "d133" = 39
  measures "d133" distance of P0 L6.end
extrude "Extrude2''''''" add sketch "Sketch3 (6)" along normal blind 5 contours L0 L2 L4 L5 L6 L7 bodies 7 in component "Divider4"
sketch "Sketch4 (4)" plane through (5, 0, 0) normal (-1, 0, 0) x (0, 0, 1) in component "Divider4"
  line L0 (5, 195) -> (5, 5)
  line L1 (5, 5) -> (10, 5)
  line L2 (10, 5) -> (10, 195)
  line L3 (10, 195) -> (5, 195)
  line L4 (5, 117) -> (10, 117)
  line L5 (10, 117) -> (10, 78)
  line L6 (10, 78) -> (5, 78)
  line L7 (5, 78) -> (5, 117)
  point P0 (5, 117)
  point P1 (10, 78)
extrude "Extrude3'''" add sketch "Sketch4 (4)" along normal blind 5 contours L0 L2 L4 L5 L6 L7 bodies 7 in component "Divider4"
sketch "Sketch5 (4)" plane through (0, 5, 0) normal (0, -1, 0) x (1, 0, 0) in component "Divider4"
  line L0 (5, 5) -> (80, 5)
  line L1 (80, 5) -> (80, 10)
  line L2 (80, 10) -> (5, 10)
  line L3 (5, 10) -> (5, 5)
  line L4 (17.5, 10) -> (67.5, 10)
  line L5 (67.5, 10) -> (67.5, 5)
  line L6 (67.5, 5) -> (17.5, 5)
  line L7 (17.5, 5) -> (17.5, 10)
  point P0 (17.5, 10)
  point P1 (67.5, 5)
extrude "Extrude4'''" add sketch "Sketch5 (4)" along normal blind 5 contours L0 L2 L4 L5 L6 L7 bodies 7 in component "Divider4"
move_face "OffsetFaces1" offset -5 1 faces at (30, 195, 8.3333) on bodies 7 in component "Divider4"
sketch "Sketch7 (2)" plane through (85, 0, 0) normal (1, 0, 0) x (0, 0, -1) in component "Divider2"
  line L0 (-85, 117) -> (-80, 117)
  line L1 (-80, 117) -> (-80, 78)
  line L2 (-80, 78) -> (-85, 78)
  line L3 (-85, 78) -> (-85, 117)
  line L4 (-50, 5) -> (-5, 5)
  line L5 (-5, 5) -> (-5, 39)
  line L6 (-5, 39) -> (0, 39)
  line L7 (0, 39) -> (0, 78)
  line L8 (0, 78) -> (-5, 78)
  line L9 (-5, 78) -> (-5, 117)
  line L10 (-5, 117) -> (0, 117)
  line L11 (0, 117) -> (0, 156)
  line L12 (0, 156) -> (-5, 156)
  line L13 (-5, 156) -> (-5, 195)
  line L14 (-5, 195) -> (-145, 195)
  line L15 (-145, 195) -> (-145, 156)
  line L16 (-145, 156) -> (-150, 156)
  line L17 (-150, 156) -> (-150, 117)
  line L18 (-150, 117) -> (-145, 117)
  line L19 (-145, 117) -> (-145, 78)
  line L20 (-145, 78) -> (-150, 78)
  line L21 (-150, 78) -> (-150, 39)
  line L22 (-150, 39) -> (-145, 39)
  line L23 (-145, 39) -> (-145, 5)
  line L24 (-145, 5) -> (-100, 5)
  line L25 (-100, 5) -> (-100, 0)
  line L26 (-100, 0) -> (-50, 0)
  line L27 (-50, 0) -> (-50, 5)
  line L28 (-100, 195) -> (-50, 195)
  line L29 (-50, 195) -> (-50, 190)
  line L30 (-50, 190) -> (-100, 190)
  line L31 (-100, 190) -> (-100, 195)
  point P0 (-100, 195)
  point P1 (-50, 190)
extrude "Extrude6'" cut sketch "Sketch7 (2)" against normal blind 5 contours L14 L28 L29 L30 L31 bodies 5 in component "Divider2"
sketch "Sketch1 (8)" plane through (0, 195, 0) normal (0, 1, 0) x (-1, 0, 0) in component "Top"
  line L0 (-80, 50) -> (-85, 50)
  line L1 (-85, 50) -> (-85, 5)
  line L2 (-85, 5) -> (-80, 5)
  line L3 (-80, 5) -> (-80, 50)
  line L4 (-85, 100) -> (-80, 100)
  line L5 (-80, 100) -> (-80, 145)
  line L6 (-80, 145) -> (-85, 145)
  line L7 (-85, 145) -> (-85, 100)
  line L8 (-5, 150) -> (-295, 150)
  line L9 (-295, 150) -> (-295, 145)
  line L10 (-295, 145) -> (-5, 145)
  line L11 (-5, 145) -> (-5, 150)
  line L12 (0, 145) -> (0, 150)
  line L13 (0, 150) -> (-5, 150)
  line L14 (-5, 150) -> (-5, 145)
  line L15 (-5, 145) -> (0, 145)
  line L16 (0, 50) -> (0, 100)
  line L17 (0, 100) -> (-5, 100)
  line L18 (-5, 100) -> (-5, 50)
  line L19 (-5, 50) -> (0, 50)
  line L20 (0, 0) -> (0, 5)
  line L21 (0, 5) -> (-5, 5)
  line L22 (-5, 5) -> (-5, 0)
  line L23 (-5, 0) -> (0, 0)
  line L24 (-295, 0) -> (-5, 0)
  line L25 (-5, 0) -> (-5, 5)
  line L26 (-5, 5) -> (-295, 5)
  line L27 (-295, 5) -> (-295, 0)
  line L28 (0, 0) -> (-85, 0)
  line L29 (-85, 0) -> (-85, 150)
  line L30 (-85, 150) -> (0, 150)
  line L31 (0, 150) -> (0, 0)
  point P0 (-85, 150)
extrude "Extrude1'''''''" add sketch "Sketch1 (8)" against normal blind 5 separate body contours L0 L3 L4 L5 L10 L15 L17 L18 L19 L21 L26 L29 L31 makes body 8 in component "Top"
sketch "Sketch2 (8)" plane through (0, 195, 0) normal (0, 1, 0) x (-1, 0, 0) in component "Top"
  line L0 (0, 145) -> (-80, 145)
  line L1 (-80, 145) -> (-80, 100)
  line L2 (-80, 100) -> (-85, 100)
  line L3 (-85, 100) -> (-85, 50)
  line L4 (-85, 50) -> (-80, 50)
  line L5 (-80, 50) -> (-80, 5)
  line L6 (-80, 5) -> (0, 5)
  line L7 (0, 5) -> (0, 50)
  line L8 (0, 50) -> (-5, 50)
  line L9 (-5, 50) -> (-5, 100)
  line L10 (-5, 100) -> (0, 100)
  line L11 (0, 100) -> (0, 145)
  circle A0 centre (-42.5, 42.5) radius 25
  dimension "d145" = 50
  dimension "d146" = 37.5
  dimension "d147" = 37.5
  measures "d145" diameter of A0
  measures "d146" distance of L6 A0.centre
  measures "d147" distance of L9 A0.centre
extrude "Extrude2'''''''" cut sketch "Sketch2 (8)" against normal blind 5 contours A0 bodies 8 in component "Top"
extrude "Extrude7" add 2 faces at (298.3333, 190, 115) (298.3333, 190, 35) along direction (0, 1, 0) blind 5 on bodies 1 bodies 1 in component "Right"
sketch "Left" plane through (0, 0, 0) normal (-1, 0, 0) x (0, 0, 1)
  line L0 (85, 117) -> (85, 78)
  line L1 (85, 78) -> (80, 78)
  line L2 (80, 78) -> (80, 117)
  line L3 (80, 117) -> (85, 117)
  line L4 (0, 78) -> (5, 78)
  line L5 (5, 78) -> (5, 39)
  line L6 (5, 39) -> (0, 39)
  line L7 (0, 39) -> (0, 5)
  line L8 (0, 5) -> (50, 5)
  line L9 (50, 5) -> (50, 0)
  line L10 (50, 0) -> (100, 0)
  line L11 (100, 0) -> (100, 5)
  line L12 (100, 5) -> (150, 5)
  line L13 (150, 5) -> (150, 39)
  line L14 (150, 39) -> (145, 39)
  line L15 (145, 39) -> (145, 78)
  line L16 (145, 78) -> (150, 78)
  line L17 (150, 78) -> (150, 117)
  line L18 (150, 117) -> (145, 117)
  line L19 (145, 117) -> (145, 156)
  line L20 (145, 156) -> (150, 156)
  line L21 (150, 156) -> (150, 195)
  line L22 (150, 195) -> (145, 195)
  line L23 (145, 195) -> (145, 190)
  line L24 (145, 190) -> (100, 190)
  line L25 (100, 190) -> (100, 195)
  line L26 (100, 195) -> (50, 195)
  line L27 (50, 195) -> (50, 190)
  line L28 (50, 190) -> (5, 190)
  line L29 (5, 190) -> (5, 195)
  line L30 (5, 195) -> (0, 195)
  line L31 (0, 195) -> (0, 156)
  line L32 (0, 156) -> (5, 156)
  line L33 (5, 156) -> (5, 117)
  line L34 (5, 117) -> (0, 117)
  line L35 (0, 117) -> (0, 78)
sketch "Front" plane through (0, 0, 150) normal (0, 0, 1) x (1, 0, 0)
  line L0 (85, 117) -> (80, 117)
  line L1 (80, 117) -> (80, 156)
  line L2 (80, 156) -> (85, 156)
  line L3 (85, 156) -> (85, 117)
  line L4 (85, 78) -> (85, 39)
  line L5 (85, 39) -> (80, 39)
  line L6 (80, 39) -> (80, 78)
  line L7 (80, 78) -> (85, 78)
  line L8 (50, 5) -> (50, 0)
  line L9 (50, 0) -> (100, 0)
  line L10 (100, 0) -> (100, 5)
  line L11 (100, 5) -> (150, 5)
  line L12 (150, 5) -> (150, 0)
  line L13 (150, 0) -> (200, 0)
  line L14 (200, 0) -> (200, 5)
  line L15 (200, 5) -> (250, 5)
  line L16 (250, 5) -> (250, 0)
  line L17 (250, 0) -> (295, 0)
  line L18 (295, 0) -> (295, 39)
  line L19 (295, 39) -> (300, 39)
  line L20 (300, 39) -> (300, 78)
  line L21 (300, 78) -> (295, 78)
  line L22 (295, 78) -> (295, 117)
  line L23 (295, 117) -> (300, 117)
  line L24 (300, 117) -> (300, 156)
  line L25 (300, 156) -> (295, 156)
  line L26 (295, 156) -> (295, 195)
  line L27 (295, 195) -> (5, 195)
  line L28 (5, 195) -> (5, 156)
  line L29 (5, 156) -> (0, 156)
  line L30 (0, 156) -> (0, 117)
  line L31 (0, 117) -> (5, 117)
  line L32 (5, 117) -> (5, 78)
  line L33 (5, 78) -> (0, 78)
  line L34 (0, 78) -> (0, 39)
  line L35 (0, 39) -> (5, 39)
  line L36 (5, 39) -> (5, 5)
  line L37 (5, 5) -> (50, 5)
sketch "Back" plane through (0, 0, 0) normal (0, 0, -1) x (-1, 0, 0)
  line L0 (-85, 117) -> (-85, 156)
  line L1 (-85, 156) -> (-80, 156)
  line L2 (-80, 156) -> (-80, 117)
  line L3 (-80, 117) -> (-85, 117)
  line L4 (-80, 39) -> (-85, 39)
  line L5 (-85, 39) -> (-85, 78)
  line L6 (-85, 78) -> (-80, 78)
  line L7 (-80, 78) -> (-80, 39)
  line L8 (-295, 39) -> (-295, 0)
  line L9 (-295, 0) -> (-250, 0)
  line L10 (-250, 0) -> (-250, 5)
  line L11 (-250, 5) -> (-200, 5)
  line L12 (-200, 5) -> (-200, 0)
  line L13 (-200, 0) -> (-150, 0)
  line L14 (-150, 0) -> (-150, 5)
  line L15 (-150, 5) -> (-100, 5)
  line L16 (-100, 5) -> (-100, 0)
  line L17 (-100, 0) -> (-50, 0)
  line L18 (-50, 0) -> (-50, 5)
  line L19 (-50, 5) -> (-5, 5)
  line L20 (-5, 5) -> (-5, 39)
  line L21 (-5, 39) -> (0, 39)
  line L22 (0, 39) -> (0, 78)
  line L23 (0, 78) -> (-5, 78)
  line L24 (-5, 78) -> (-5, 117)
  line L25 (-5, 117) -> (0, 117)
  line L26 (0, 117) -> (0, 156)
  line L27 (0, 156) -> (-5, 156)
  line L28 (-5, 156) -> (-5, 195)
  line L29 (-5, 195) -> (-295, 195)
  line L30 (-295, 195) -> (-295, 156)
  line L31 (-295, 156) -> (-300, 156)
  line L32 (-300, 156) -> (-300, 117)
  line L33 (-300, 117) -> (-295, 117)
  line L34 (-295, 117) -> (-295, 78)
  line L35 (-295, 78) -> (-300, 78)
  line L36 (-300, 78) -> (-300, 39)
  line L37 (-300, 39) -> (-295, 39)
sketch "Top" plane through (0, 195, 0) normal (0, 1, 0) x (-1, 0, 0)
  circle A0 centre (-42.5, 42.5) radius 25
  line L0 (0, 145) -> (-80, 145)
  line L1 (-80, 145) -> (-80, 100)
  line L2 (-80, 100) -> (-85, 100)
  line L3 (-85, 100) -> (-85, 50)
  line L4 (-85, 50) -> (-80, 50)
  line L5 (-80, 50) -> (-80, 5)
  line L6 (-80, 5) -> (0, 5)
  line L7 (0, 5) -> (0, 50)
  line L8 (0, 50) -> (-5, 50)
  line L9 (-5, 50) -> (-5, 100)
  line L10 (-5, 100) -> (0, 100)
  line L11 (0, 100) -> (0, 145)
sketch "Sketch3 (7)" plane through (85, 0, 0) normal (1, 0, 0) x (0, 0, -1) in component "Top"
  line L0 (-100, 190) -> (-100, 195)
  line L1 (-100, 195) -> (-145, 195)
  line L2 (-145, 195) -> (-145, 156)
  line L3 (-145, 156) -> (-150, 156)
  line L4 (-150, 156) -> (-150, 117)
  line L5 (-150, 117) -> (-145, 117)
  line L6 (-145, 117) -> (-145, 78)
  line L7 (-145, 78) -> (-150, 78)
  line L8 (-150, 78) -> (-150, 39)
  line L9 (-150, 39) -> (-145, 39)
  line L10 (-145, 39) -> (-145, 5)
  line L11 (-145, 5) -> (-100, 5)
  line L12 (-100, 5) -> (-100, 0)
  line L13 (-100, 0) -> (-50, 0)
  line L14 (-50, 0) -> (-50, 5)
  line L15 (-50, 5) -> (-5, 5)
  line L16 (-5, 5) -> (-5, 39)
  line L17 (-5, 39) -> (0, 39)
  line L18 (0, 39) -> (0, 78)
  line L19 (0, 78) -> (-5, 78)
  line L20 (-5, 78) -> (-5, 117)
  line L21 (-5, 117) -> (0, 117)
  line L22 (0, 117) -> (0, 156)
  line L23 (0, 156) -> (-5, 156)
  line L24 (-5, 156) -> (-5, 195)
  line L25 (-5, 195) -> (-50, 195)
  line L26 (-50, 195) -> (-50, 190)
  line L27 (-50, 190) -> (-100, 190)
  line L28 (-85, 117) -> (-80, 117)
  line L29 (-80, 117) -> (-80, 78)
  line L30 (-80, 78) -> (-85, 78)
  line L31 (-85, 78) -> (-85, 117)
sketch "Sketch4 (5)" plane through (85, 0, 0) normal (1, 0, 0) x (0, 0, -1) in component "Top"
  line L0 (-100, 190) -> (-100, 195)
  line L1 (-100, 195) -> (-145, 195)
  line L2 (-145, 195) -> (-145, 156)
  line L3 (-145, 156) -> (-150, 156)
  line L4 (-150, 156) -> (-150, 117)
  line L5 (-150, 117) -> (-145, 117)
  line L6 (-145, 117) -> (-145, 78)
  line L7 (-145, 78) -> (-150, 78)
  line L8 (-150, 78) -> (-150, 39)
  line L9 (-150, 39) -> (-145, 39)
  line L10 (-145, 39) -> (-145, 5)
  line L11 (-145, 5) -> (-100, 5)
  line L12 (-100, 5) -> (-100, 0)
  line L13 (-100, 0) -> (-50, 0)
  line L14 (-50, 0) -> (-50, 5)
  line L15 (-50, 5) -> (-5, 5)
  line L16 (-5, 5) -> (-5, 39)
  line L17 (-5, 39) -> (0, 39)
  line L18 (0, 39) -> (0, 78)
  line L19 (0, 78) -> (-5, 78)
  line L20 (-5, 78) -> (-5, 117)
  line L21 (-5, 117) -> (0, 117)
  line L22 (0, 117) -> (0, 156)
  line L23 (0, 156) -> (-5, 156)
  line L24 (-5, 156) -> (-5, 195)
  line L25 (-5, 195) -> (-50, 195)
  line L26 (-50, 195) -> (-50, 190)
  line L27 (-50, 190) -> (-100, 190)
  line L28 (-85, 117) -> (-80, 117)
  line L29 (-80, 117) -> (-80, 78)
  line L30 (-80, 78) -> (-85, 78)
  line L31 (-85, 78) -> (-85, 117)